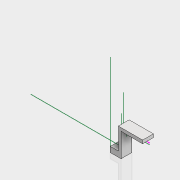
# Autodesk Inventor part: ЛЦМК000002.00.00.00.00.07
Saved by Autodesk Inventor 2021.2 (Build 252289000, 289)
## iProperties
Created: 2025-10-26
Part Number: ЛЦМК000002.00.00.00.00.07
Material: Generic
Document SubType Name: Modeling
Designer: Захаров
Density: 1 g/cm^3
Appearance: Default
Author: Захаров
Autodesk Inventor part; units mm, degrees
ref_plane "YZ Plane" through (0, 0, 0) normal (1, 0, 0) x (0, 1, 0)
ref_plane "XZ Plane" through (0, 0, 0) normal (0, 1, 0) x (-1, 0, 0)
ref_plane "XY Plane" through (0, 0, 0) normal (0, 0, 1) x (1, 0, 0)
sketch "Sketch2" plane through (0, 0, 0) normal (0, 0, 1) x (1, 0, 0)
  line L0 (-17.5, -21) -> (-7.5, -21) projected
  line L1 (-91.1, -16) -> (-5.5, -16) projected
  line L2 (-5.5, -16) -> (-5.5, 28.3) projected
  line L3 (-12.5, -21) -> (-12.5, -16)
  line L4 (-12.5, -21) -> (-2.5, -21)
  line L5 (-2.5, -21) -> (-2.5, -15.999)
  line L6 (-2.5, -15.999) -> (-12.5, -15.999)
  line L7 (-12.5, -15.999) -> (-12.5, -21)
  line L8 (-2.5, -15.999) -> (-5.0122, -15.999)
  line L9 (-5.0122, -15.999) -> (-5.0122, 4.001)
  line L10 (-5.0122, 4.001) -> (-2.5, 4.001)
  line L11 (-2.5, 4.001) -> (-2.5, -15.999)
  line L12 (-2.5, 4.001) -> (17.5, 4.001)
  line L13 (17.5, 4.001) -> (17.5, 1.001)
  line L14 (17.5, 1.001) -> (-2.5, 1.001)
  line L15 (-2.5, 1.001) -> (-2.5, 4.001)
  arc A0 (23.0689, 0.2342) -> (17.5, 4.001) centre (17.5, -1.999) ccw
  arc A1 (21.9703, 0.2342) -> (20.0013, 1.001) centre (20.0013, -1.9105) ccw
  line L16 (20.0013, 1.001) -> (17.5, 1.001)
  line L17 (23.0689, 0.2342) -> (21.9703, 0.2342)
  point P0 (0, 0)
  point P1 (-5.5, -15.999)
  dimension "d0" = 10
  dimension "d1" = 20
  dimension "d2" = 20
  dimension "d3" = 3
  dimension "d9" = 6
  constraints: 30 end point, 6 parallel, 5 horizontal, 4 perpendicular, 4 point on circle, 2 centre point, 1 midpoint, 1 point on line, 1 tangent
  measures "d0" distance of L6.end L5.end
  measures "d1" distance of L8.end L9.end
  measures "d2" distance of L13.end L14.end
  measures "d3" distance of L13.end L12.end
  measures "d9" radius of A0
extrude "Extrusion1" add sketch "Sketch2" against normal mid plane 10
sketch "Sketch3" plane through (-12.5, -21, -5) normal (0, -1, 0) x (1, 0, 0)
  line L0 (5, 0) -> (5, -5) projected
  line L1 (0, 0) -> (7.4878, 0) projected
  arc A0 (2.7054, 10) -> (2.7054, 0) centre (6.0221, 5) ccw
  line L2 (2.7054, 0) -> (-2.2946, 0)
  line L3 (0, 0) -> (0, 10) projected
  line L4 (-2.2946, 10) -> (2.7054, 10)
  line L5 (-2.2946, 0) -> (-2.2946, 10)
  point P0 (12.5, 5)
  point P1 (2.7054, 0)
  dimension "d6" = 6
  constraints: 6 end point, 2 point on circle, 1 centre point, 1 collinear, 1 perpendicular, 1 vertical
  measures "d6" radius of A0
extrude "Extrusion2" cut sketch "Sketch3" against normal blind 10 contours L3 L4 A0 L1
body "Solid1"
